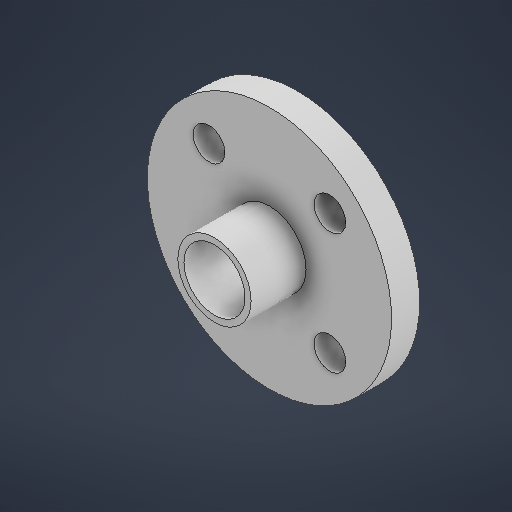
# Autodesk Inventor part: SAFRS-P-0013
Saved by Autodesk Inventor 2026.2 (Build 302298000, 298)
## iProperties
Created: 2025-11-21
Part Number: SAFRS-P-0013
Material: 일반
Document SubType Name: Modeling
Designer: jaewook
Density: 1 g/cm^3
Appearance: 기본값
Author: jaewook
Title: Pitch Motor V1
Autodesk Inventor part; units mm, degrees
ref_plane "YZ Plane" through (0, 0, 0) normal (1, 0, 0) x (0, 1, 0)
ref_plane "XZ Plane" through (0, 0, 0) normal (0, 1, 0) x (-1, 0, 0)
ref_plane "XY Plane" through (0, 0, 0) normal (0, 0, 1) x (1, 0, 0)
sketch "스케치1" plane through (0, 0, 0) normal (0, 0, 1) x (1, 0, 0)
  circle A0 centre (0.4717, -6.8619) radius 1.3
  circle A1 centre (0.4717, 3.0376) radius 1.3
  circle A2 centre (-9.4278, 3.0376) radius 1.3
  circle A3 centre (-9.4278, -6.8619) radius 1.3
  circle A4 centre (-4.4781, -1.9122) radius 10
  circle A5 centre (-4.4781, -1.9122) radius 5.5
  circle A6 centre (-4.4781, -1.9122) radius 10 projected
  circle A7 centre (0.4717, -6.8619) radius 1.3 projected
  circle A8 centre (0.4717, 3.0376) radius 1.3 projected
  circle A9 centre (-9.4278, 3.0376) radius 1.3 projected
  circle A10 centre (-9.4278, -6.8619) radius 1.3 projected
  point P0 (0, 0)
  dimension "d6" = 20
  dimension "d7" = 11
  dimension "d8" = 2.6
  dimension "d9" = 2.6
  dimension "d10" = 2.6
  dimension "d11" = 2.6
  constraints: 6 centre point, 6 coincident
  measures "d6" diameter of A4
  measures "d7" diameter of A5
  measures "d8" diameter of A1
  measures "d9" diameter of A0
  measures "d10" diameter of A3
  measures "d11" diameter of A2
extrude "돌출1" add sketch "스케치1" along normal blind 2.3 contours A4 | A5
sketch "스케치2" plane through (-4.4781, -1.9122, 2.3) normal (0, 0, 1) x (1, 0, 0)
  circle A0 centre (0, 0) radius 10 projected
  circle A1 centre (0, 0) radius 3
  circle A2 centre (0, 0) radius 2.5
  dimension "d2" = 6
  dimension "d5" = 5
  constraints: 2 centre point, 2 coincident
  measures "d2" diameter of A1
  measures "d5" diameter of A2
extrude "돌출2" add sketch "스케치2" along normal blind 4.5 contours A1
